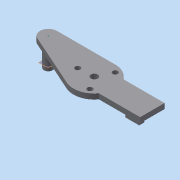
# Autodesk Inventor part: bras-Codeur
Saved by Autodesk Inventor 2016 (Build 200138000, 138)
## iProperties
Created: 2017-02-14
Part Number: bras-Codeur
Material: Generic
Document SubType Name: Modeling
Designer: Aegir
Density: 1 g/cm^3
Appearance: Default
Author: Aegir
Autodesk Inventor part; units mm, degrees
ref_plane "YZ Plane" through (0, 0, 0) normal (1, 0, 0) x (0, 1, 0)
ref_plane "XZ Plane" through (0, 0, 0) normal (0, 1, 0) x (-1, 0, 0)
ref_plane "XY Plane" through (0, 0, 0) normal (0, 0, 1) x (1, 0, 0)
sketch "Esquisse1" plane through (0, 0, 0) normal (0, 0, 1) x (1, 0, 0)
  circle A0 centre (0, 0) radius 2.5 projected
  circle A1 centre (33.5, -7) radius 12 projected
  circle A2 centre (33.5, -7) radius 2 projected
  circle A3 centre (38.485, -14.4933) radius 1.5 projected
  circle A4 centre (24.5181, -7.5705) radius 1.5 projected
  circle A5 centre (37.4969, 1.0638) radius 1.5 projected
  line L0 (0, 5) -> (33.5, 5)
  line L1 (29.0343, -18.1381) -> (-2.5, -4.0756)
  arc A6 (29.0343, -18.1381) -> (33.5, 5) centre (33.5, -7) ccw
  arc A7 (0, 5) -> (-2.5, -4.0756) centre (0, 0.1179) ccw
  circle A8 centre (0, 0.1179) radius 2.4972
  circle A9 centre (37.4969, 1.0638) radius 1.5
  circle A10 centre (24.5181, -7.5705) radius 1.5
  circle A11 centre (38.485, -14.4933) radius 1.5
  constraints: 6 centre point, 6 point on circle, 4 coincident, 4 concentric, 4 end point, 2 tangent, 1 horizontal
extrude "Extrusion1" add sketch "Esquisse1" along normal blind 3 contours A1 L1 | A1 L1 A7 L0 picked at (27.6177, -3.3612)
sketch "Esquisse2" plane through (0, 0, 3) normal (0, 0, 1) x (1, 0, 0)
  point P0 (0, 0)
sketch "Esquisse3" plane through (0, 0, 3) normal (0, 0, 1) x (1, 0, 0)
  line L0 (42.9839, -14.0611) -> (66.9147, -14.0611)
  line L1 (66.9147, -14.0611) -> (66.9147, 0)
  line L2 (66.9147, 0) -> (42.9839, 0)
  circle A0 centre (33.5, -7) radius 2 projected
  circle A1 centre (37.4969, 1.0638) radius 1.5 projected
  circle A2 centre (24.5181, -7.5705) radius 1.5 projected
  circle A3 centre (38.485, -14.4933) radius 1.5 projected
  arc A4 (-2.4972, 0.1179) -> (2.4972, 0.1179) centre (0, 0) ccw projected
  arc A5 (2.4972, 0.1179) -> (-2.4972, 0.1179) centre (0, 0.1179) ccw projected
  arc A6 (0, 5) -> (-2.5, -4.0756) centre (0, 0.1179) ccw projected
  line L3 (-2.5, -4.0756) -> (29.0343, -18.1381) projected
  arc A7 (29.0343, -18.1381) -> (33.5, 5) centre (33.5, -7) ccw projected
  line L4 (33.5, 5) -> (0, 5) projected
  arc A8 (42.9839, -14.0611) -> (42.9839, 0) centre (34.4207, -7.0306) ccw
  constraints: 6 end point, 2 point on circle, 1 centre point, 1 horizontal, 1 parallel, 1 perpendicular
extrude "Extrusion2" add sketch "Esquisse3" against normal blind 3 contours A8 A7 L0 | A7 L2 L1 L0 | A8 L2 A7
sketch "Esquisse4" plane through (0, 0, 0) normal (0, 0, -1) x (-1, 0, 0)
  point P0 (0, 0)
sketch "Esquisse5" plane through (0, 0, 0) normal (0, 0, -1) x (-1, 0, 0)
  line L0 (-58.7293, -9.4268) -> (-61.7293, -9.4268)
  line L1 (-61.7293, -9.4268) -> (-61.7293, -6.4268)
  line L2 (-61.7293, -6.4268) -> (-58.7293, -6.4268)
  line L3 (-58.7293, -6.4268) -> (-58.7293, -9.4268)
  point P0 (0, 0)
  dimension "d4" = 3
  dimension "d5" = 3
  constraints: 8 end point, 2 parallel, 1 horizontal, 1 perpendicular
  measures "d4" distance between parallel lines of L3 L1
  measures "d5" distance of L2.end L0.start
extrude "Extrusion3" add sketch "Esquisse5" along normal blind 4
sketch "Esquisse6" plane through (61.7293, -9.4268, 0) normal (1, 0, 0) x (0, 0, -1)
  line L0 (0, 3) -> (4, 3) projected
  line L1 (0, 0) -> (0, 3) projected
  line L2 (0, 0) -> (4, 0) projected
  line L3 (4, 3) -> (4, 0) projected
  line L4 (0, 3) -> (4, 3) projected
  line L5 (0, 0) -> (4, 0) projected
  line L6 (4, 0) -> (6, 0)
  line L7 (6, 0) -> (6, 3)
  line L8 (6, 3) -> (4, 3)
  line L9 (4, 3) -> (4, 0)
  point P0 (0, 9.4268)
  dimension "d8" = 2
  constraints: 8 end point, 2 parallel, 1 horizontal, 1 perpendicular
  measures "d8" distance of L7.end L8.end
extrude "Extrusion4" add sketch "Esquisse6" against normal blind 8 contours L8 L7 L6 L3
sketch "Esquisse8" plane through (53.7293, -6.4268, -4) normal (0, 0, 1) x (1, 0, 0)
  line L0 (5, -3) -> (5, 0) projected
  line L1 (5, 0) -> (0, 0) projected
  line L2 (0, -3) -> (0, 0) projected
  line L3 (5, -3) -> (0, -3) projected
  line L4 (0, -3) -> (0, 0) projected
  line L5 (5, 0) -> (0, 0) projected
  line L6 (0, -3) -> (1.2053, -3)
  line L7 (1.2053, -3) -> (1.2053, 0)
  line L8 (1.2053, 0) -> (0, 0)
  line L9 (0, 0) -> (0, -3)
  point P0 (-53.7293, 6.4268)
  constraints: 8 end point, 2 parallel, 1 horizontal, 1 perpendicular, 1 point on line
extrude "Extrusion5" add sketch "Esquisse8" along normal blind 1 contours L3 L2 L1 L7
sketch "Esquisse9" plane through (0, 0, 3) normal (0, 0, 1) x (1, 0, 0)
  arc A0 (-2.4972, 0.1179) -> (2.4972, 0.1179) centre (0, 0) ccw projected
  arc A1 (2.4972, 0.1179) -> (-2.4972, 0.1179) centre (0, 0.1179) ccw projected
extrude "Extrusion6" add sketch "Esquisse9" against normal blind 16
ref_plane "Plan de construction1" through (0, 0, -10.3) normal (0, 0, -1) x (-1, 0, 0)
sketch "Esquisse13" plane through (0, 0, -13) normal (0, 0, -1) x (-1, 0, 0)
  circle A0 centre (0, 0) radius 2.932
  constraints: 1 centre point, 1 coincident
extrude "Extrusion8" cut sketch "Esquisse13" against normal up to surface (2.7 mm away)
sketch "Esquisse14" plane through (0, 0, -10.3) normal (0, 0, -1) x (-1, 0, 0)
  circle A0 centre (0, 0) radius 2
  dimension "d20" = 4
  constraints: 1 centre point, 1 coincident
  measures "d20" diameter of A0
extrude "Extrusion9" add sketch "Esquisse14" along normal blind 0.6
sketch "Esquisse15" plane through (0, 0, -10.9) normal (0, 0, -1) x (-1, 0, 0)
  circle A0 centre (0, 0) radius 2.5
  constraints: 1 centre point, 1 coincident
extrude "Extrusion10" add sketch "Esquisse15" along normal blind 2
